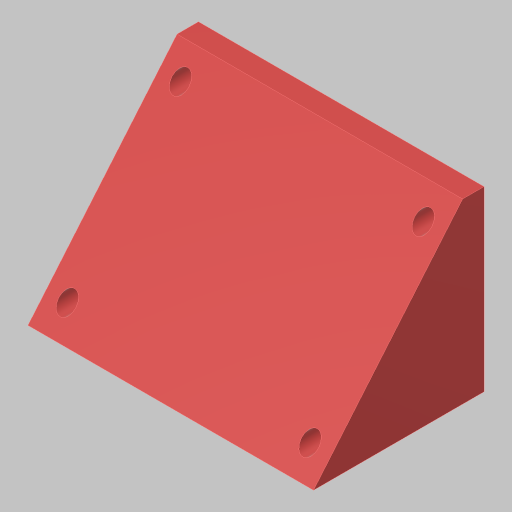
# Autodesk Inventor part: limelight mount
Saved by Autodesk Inventor 2023.5 (Build 275446000, 446)
## iProperties
Created: 2025-03-27
Part Number: limelight mount
Material: ABS Plastic
Document SubType Name: Modeling
Designer: slick
Density: 1.06 g/cm^3
Appearance: Smooth - Red
Author: slick
Autodesk Inventor part; units mm, degrees
ref_plane "YZ Plane" through (0, 0, 0) normal (1, 0, 0) x (0, 1, 0)
ref_plane "XZ Plane" through (0, 0, 0) normal (0, 1, 0) x (-1, 0, 0)
ref_plane "XY Plane" through (0, 0, 0) normal (0, 0, 1) x (1, 0, 0)
sketch "Sketch1" plane through (0, 0, 0) normal (0, 0, 1) x (1, 0, 0)
  line L0 (36, -20) -> (-36, -20) construction
  line L1 (-36, -20) -> (-36, 20) construction
  line L2 (-36, 20) -> (36, 20) construction
  line L3 (36, 20) -> (36, -20) construction
  line L4 (36, -20) -> (-36, 20) construction
  line L5 (-36, -20) -> (36, 20) construction
  line L6 (42.35, -26.35) -> (-42.35, -26.35)
  line L7 (-42.35, -26.35) -> (-42.35, 26.35)
  line L8 (-42.35, 26.35) -> (42.35, 26.35)
  line L9 (42.35, 26.35) -> (42.35, -26.35)
  line L10 (42.35, -26.35) -> (-42.35, 26.35) construction
  line L11 (-42.35, -26.35) -> (42.35, 26.35) construction
  point P0 (0, 0)
  dimension "d0" = 72
  dimension "d1" = 40
  dimension "d2" = 6.35
  dimension "d3" = 6.35
  constraints: 24 end point, 4 coincident, 4 midpoint, 4 parallel, 2 horizontal, 2 perpendicular
  measures "d0" distance of L1.end L2.end
  measures "d1" distance of L0.end L1.end
  measures "d2" distance between parallel lines of L8 L2
  measures "d3" distance between parallel lines of L1 L7
extrude "Extrusion1" add sketch "Sketch1" along normal blind 6.35
sketch "Sketch2" plane through (42.35, -26.35, 0) normal (1, 0, 0) x (0, 0, -1)
  line L0 (-6.35, 0) -> (-6.35, 52.7) projected
  line L1 (-6.35, 52.7) -> (-50.5706, 0)
  line L2 (-50.5706, 0) -> (-6.35, 0)
  point P0 (0, 26.35)
  dimension "d13" = 40
  constraints: 4 end point, 1 perpendicular
  measures "d13" angle of L0 L1
extrude "Extrusion2" add sketch "Sketch2" against normal up to surface (84.7 mm away)
hole "Hole2" at (-36, 20, 0) at (-36, -20, 0) at (36, -20, 0) at (36, 20, 0) direction (0, 0, 1) diameter 5.1054 end through all clearance for "Socket Head Cap Screw" size "#10" standard "Ansi Unified Screw Threads"
body "Solid1"
